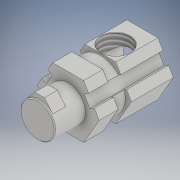
# Autodesk Inventor part: дз2 2
Saved by Autodesk Inventor 2019.3 (Build 233278000, 278)
## iProperties
Created: 2020-03-25
Part Number: дз2 2
Material: Типовые
Document SubType Name: Modeling
Designer: Admin
Density: 1 g/cm^3
Appearance: По умолчанию
Author: Admin
Autodesk Inventor part; units mm, degrees
ref_plane "YZ Plane" through (0, 0, 0) normal (1, 0, 0) x (0, 1, 0)
ref_plane "XZ Plane" through (0, 0, 0) normal (0, 1, 0) x (-1, 0, 0)
ref_plane "XY Plane" through (0, 0, 0) normal (0, 0, 1) x (1, 0, 0)
sketch "Эскиз1" plane through (0, 0, 0) normal (0, 0, 1) x (1, 0, 0)
  line L0 (-4.0415, -7) -> (-8.0829, 0)
  line L1 (-8.0829, 0) -> (-4.0415, 7)
  line L2 (-4.0415, 7) -> (4.0415, 7)
  line L3 (4.0415, 7) -> (8.0829, 0)
  line L4 (8.0829, 0) -> (4.0415, -7)
  line L5 (4.0415, -7) -> (-4.0415, -7)
  point P0 (0, 0)
  point P1 (0, 0)
  dimension "d0" = 14
  constraints: 12 end point, 1 coincident, 1 horizontal alignment, 13 other
  measures "d0" distance between parallel lines of L5 L2
extrude "Выдавливание1" add sketch "Эскиз1" along normal blind 19.4
sketch "Эскиз2" plane through (0, 0, 19.4) normal (0, 0, 1) x (1, 0, 0)
  circle A0 centre (0, 0) radius 4.5
  dimension "d3" = 9
  constraints: 1 centre point, 1 coincident
  measures "d3" diameter of A0
extrude "Выдавливание2" add sketch "Эскиз2" along normal blind 8
sketch "Эскиз3" plane through (0, 0, 0) normal (0, 0, -1) x (-1, 0, 0)
  line L0 (-4.0415, -7) -> (4.0415, -7) projected
  point P0 (0, 0)
  point P1 (0, -0.675)
  dimension "d6" = 6.325
  measures "d6" distance from line of L0 point (0, -0.675)
hole "Отверстие1" at (0, -0.675, 0) direction (0, 0, 1) diameter 9.95 depth 18 tip angle 120
sketch "Эскиз4" plane through (0, 0, 0) normal (0, 0, -1) x (-1, 0, 0)
  line L0 (-6.8329, 2.1651) -> (-5.6529, 1.4838)
  line L1 (-5.6529, 1.4838) -> (-4.1529, 4.0819)
  line L2 (-4.1529, 4.0819) -> (-5.3329, 4.7631)
  line L3 (-4.0415, 7) -> (-8.0829, 0) projected
  line L4 (6.8329, 2.1651) -> (5.6529, 1.4838)
  line L5 (5.6529, 1.4838) -> (4.1529, 4.0819)
  line L6 (4.1529, 4.0819) -> (5.3329, 4.7631)
  line L7 (-5.3413, 0.0236) -> (-2.2117, 5.4442)
  line L8 (5.3329, 4.7631) -> (6.8329, 2.1651)
  point P0 (0, 0)
  dimension "d14" = 3
  dimension "d15" = 2.5
  dimension "d18" = 1
  constraints: 16 end point, 2 parallel
  measures "d14" distance of L0.end L1.end
  measures "d15" distance of L3.end L0.start
  measures "d18" distance between parallel lines of L7 L1
extrude "Выдавливание3" cut sketch "Эскиз4" against normal through all
sketch "Эскиз5" plane through (0, 0, 0) normal (1, 0, 0) x (0, 1, 0)
  line L0 (-6.5, 14.4) -> (-6.5, 11)
  line L1 (-6.5, 11) -> (-15.5512, 11)
  line L2 (-15.5512, 11) -> (-15.5512, 14.4)
  line L3 (-15.5512, 14.4) -> (-6.5, 14.4)
  line L4 (0, 0) -> (0, 19.4) projected
  line L5 (-7, 19.4) -> (0, 19.4) projected
  line L6 (0, 0) -> (-7, 0) projected
  line L7 (0, -5.48) -> (0, 32.88) projected
  dimension "d21" = 6.5
  dimension "d22" = 5
  dimension "d23" = 11
  constraints: 8 end point, 2 horizontal, 2 vertical
  measures "d21" distance between parallel lines of L4 L0
  measures "d22" distance between parallel lines of L5 L3
  measures "d23" distance between parallel lines of L6 L1
revolve "Вращение1" cut sketch "Эскиз5" angle 360 about axis through (0, 0, -10) along (0, 0, 1)
sketch "Эскиз6" plane through (-4.0415, 7, 0) normal (0, 1, 0) x (1, 0, 0)
  circle A0 centre (4.0415, -7) radius 3.75
  line L0 (0, 0) -> (8.0829, 0) projected
  point P0 (4.0415, 0)
  point P1 (4.0415, 0)
  dimension "d25" = 7.5
  dimension "d26" = 7
  constraints: 1 centre point, 1 midpoint, 1 vertical alignment
  measures "d25" diameter of A0
  measures "d26" distance of point (4.041, 0) A0.centre
extrude "Выдавливание4" cut sketch "Эскиз6" against normal up to next
thread "Резьба1" size "M8x1.25" class "6H" standard "ANSI Metric M Profile" full length
ref_plane "РабПлоскость1" through (0, 0, 26.9) normal (0, 0, 1) x (1, 0, 0)
sketch "Эскиз7" plane through (0, 0, 26.9) normal (0, 0, 1) x (1, 0, 0)
  line L0 (-1.2214, 5.5) -> (1.2786, 5.5)
  circle A0 centre (0, 0) radius 4.5 projected
  line L1 (-1.2214, 5.5) -> (-3.4225, 2.9218)
  circle A1 centre (0, 0) radius 4.5 projected
  line L2 (1.2786, 5.5) -> (3.4597, 2.8775)
  arc A2 (-3.4225, 2.9218) -> (0, 4.5) centre (0, 0) ccw
  dimension "d32" = 2.5
  dimension "d33" = 5.5
  constraints: 6 end point, 5 point on circle, 2 tangent, 1 centre point, 1 concentric, 1 horizontal, 3 other
  measures "d32" distance of L0.start L0.end
  measures "d33" distance from line of point (0, 0) L0
extrude "Выдавливание5" add sketch "Эскиз7" against normal blind 3.4
chamfer "Фаска1" distance 0.1 angle 45 1 edges at (-3.75, 7, 7)
chamfer "Фаска2" distance 0.2 angle 45 1 edges at (-4.5, 0, 27.4)
